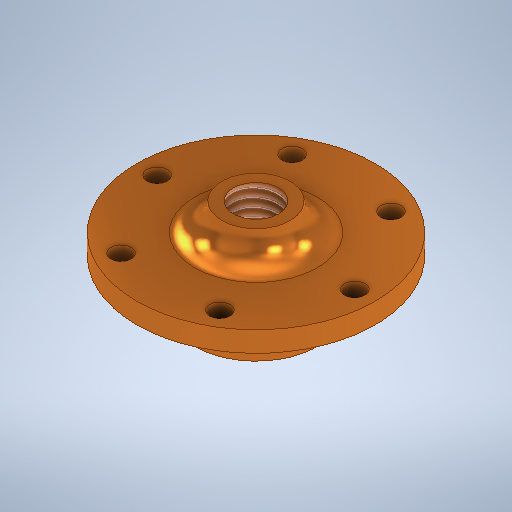
# Autodesk Inventor part: 156
Saved by Autodesk Inventor 2025.1 (Build 291241000, 241)
## iProperties
Created: 2024-08-03
Part Number: 156
Material: Gold
Document SubType Name: Modeling
Designer: ffogue
Density: 19.3 g/cm^3
Appearance: Metal 1600F Hot
Author: ffogue
Autodesk Inventor part; units mm, degrees
ref_plane "XZ Plane" through (0, 0, 0) normal (0, 1, 0) x (-1, 0, 0)
ref_plane "XY Plane" through (0, 0, 0) normal (0, 0, 1) x (1, 0, 0)
ref_plane "Work Plane1" through (0, 0, 0) normal (1, 0, 0) x (0, 1, 0)
sketch "Sketch3" plane through (0, 0, 0) normal (1, 0, 0) x (0, 1, 0)
  line L0 (0, 0) -> (0, 14)
  line L1 (0, 14) -> (-5, 14)
  arc A0 (-9, 10) -> (-5, 14) centre (-9, 14) ccw
  line L2 (-9, 10) -> (-17.5, 10)
  line L3 (-17.5, 10) -> (-17.5, 7)
  line L4 (-17.5, 7) -> (-9, 7)
  line L5 (-9, 7) -> (-9, 0)
  line L6 (-9, 0) -> (0, 0)
  dimension "d10" = 4
  dimension "d11" = 3
  dimension "d12" = 35
  dimension "d13" = 7
  dimension "d14" = 18
  constraints: 14 end point, 4 perpendicular, 2 point on circle, 2 vertical alignment, 1 centre point, 1 horizontal, 1 parallel, 1 point on line, 1 tangent
  measures "d10" radius of A0
  measures "d11" distance of L2.end L3.end
  measures "d12" diameter of L3 L0
  measures "d13" distance of L4.end L5.end
  measures "d14" diameter of L5 L0
revolve "Revolution2" add sketch "Sketch3" angle 360 about axis through (0, 0, 0) along (0, 0, 1)
sketch "Sketch4" plane through (0, 0, 14) normal (0, 0, 1) x (1, 0, 0)
  circle A0 centre (0, 0) radius 5 projected
  point P0 (0, 0)
  constraints: 1 coincident
hole "Hole1" at (0, 0, 14) direction (0, 0, -1) diameter 6.647 depth 8 thread size "M8x1.25" class "6H" standard "ISO Metric profile"
sketch "Sketch5" plane through (0, 0, 0) normal (0, 0, -1) x (-1, 0, 0)
  circle A0 centre (0, 0) radius 9 projected
  point P0 (0, 0)
  constraints: 1 coincident
hole "Hole2" at (0, 0, 0) direction (0, 0, 1) diameter 5 depth 6
sketch "Sketch6" plane through (0, 0, 10) normal (0, 0, 1) x (1, 0, 0)
  line L0 (0, 0) -> (0, 20.3424) construction
  circle A0 centre (0, 0) radius 2.5 projected
  line L1 (0, 0) -> (-11.8721, 20.5631) construction
  circle A1 centre (0, 0) radius 5 projected
  circle A2 centre (0, 0) radius 14.5 construction
  point P0 (-7.25, 12.5574)
  dimension "d31" = 29
  dimension "d30" = 30
  constraints: 4 end point, 1 coincident, 1 point on line, 1 vertical, 3 other
  measures "d30" angle of L0 L1
hole "Hole3" at (-7.25, 12.5574, 10) direction (0, 0, -1) diameter 3 depth 3
pattern_circular "Circular Pattern1" count 6 over 360 about axis through (0, 0, 8.5) along (0, 0, 1) of "Hole3"
body "Solid2"
